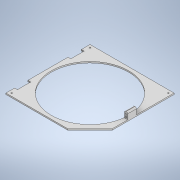
# Autodesk Inventor part: Box_Walls_2
Saved by Autodesk Inventor 2022 (Build 260153000, 153)
## iProperties
Created: 2023-02-27
Part Number: Box_Walls_2
Material: Generic
Document SubType Name: Modeling
Designer: zarek
Density: 1 g/cm^3
Appearance: Default
Author: zarek
Autodesk Inventor part; units mm, degrees
ref_plane "YZ Plane" through (0, 0, 0) normal (1, 0, 0) x (0, 1, 0)
ref_plane "XZ Plane" through (0, 0, 0) normal (0, 1, 0) x (-1, 0, 0)
ref_plane "XY Plane" through (0, 0, 0) normal (0, 0, 1) x (1, 0, 0)
sketch "Sketch1" plane through (0, 0, 0) normal (0, 1, 0) x (-1, 0, 0)
  line L0 (101.6, -101.6) -> (-101.6, -101.6)
  line L1 (-101.6, -101.6) -> (-101.6, 101.6)
  line L2 (-101.6, 101.6) -> (101.6, 101.6)
  line L3 (101.6, 101.6) -> (101.6, -101.6)
  line L4 (96.6, -96.6) -> (-96.6, -96.6)
  line L5 (-96.6, -96.6) -> (-96.6, 96.6)
  line L6 (-96.6, 96.6) -> (96.6, 96.6)
  line L7 (96.6, 96.6) -> (96.6, -96.6)
  line L8 (101.6, 101.6) -> (-40.4, 101.6)
  circle A0 centre (0, 0) radius 88.9
  circle A1 centre (0, 0) radius 109.3376
  line L9 (-40.4, 101.6) -> (-101.6, 40.4)
  line L10 (-45.4, 101.6) -> (-101.6, 45.4)
  line L11 (96.6, 96.6) -> (96.6, 101.6)
  line L12 (-45.4, 101.6) -> (-35.4, 101.6)
  line L13 (-35.4, 101.6) -> (-35.4, 96.6)
  line L14 (-35.4, 96.6) -> (-45.4, 96.6)
  line L15 (-45.4, 96.6) -> (-45.4, 101.6)
  circle A2 centre (0, 0) radius 111.3376
  point P0 (96.6, 51.2168)
  point P1 (101.6, 40.4)
  point P2 (101.6, -40.4)
  point P3 (96.6, -51.2168)
  point P4 (-96.6, 45.4)
  point P5 (-45.4, 96.6)
  dimension "d0" = 203.2
  dimension "d1" = 203.2
  dimension "d2" = 101.6
  dimension "d3" = 101.6
  dimension "d4" = 5
  dimension "d5" = 5
  dimension "d6" = 5
  dimension "d7" = 5
  dimension "d10" = 142
  dimension "d12" = 61.2
  dimension "d14" = 177.8
  dimension "d15" = 5
  dimension "d16" = 5
  dimension "d17" = 10
  dimension "d34" = 2
  constraints: 32 end point, 7 parallel, 6 point on line, 4 perpendicular, 3 centre point, 3 coincident, 3 horizontal, 2 point on circle
  measures "d0" distance between parallel lines of L2 L0
  measures "d1" distance between parallel lines of L1 L3
  measures "d2" distance from line of L0 point (0, 0)
  measures "d3" distance from line of L1 point (0, 0)
  measures "d4" distance between parallel lines of L4 L0
  measures "d5" distance between parallel lines of L1 L5
  measures "d6" distance between parallel lines of L2 L6
  measures "d7" distance between parallel lines of L3 L7
  measures "d10" distance of L2.end L8.end
  measures "d12" distance from line of L1 L8.end
  measures "d14" diameter of A0
  measures "d15" distance of L10.end L9.end
  measures "d16" distance of L10.start L8.end
  measures "d17" distance of L13.end L14.end
  measures "d34" radial gap between concentric circles of A1 A2
extrude "Extrusion1" add sketch "Sketch1" along normal blind 3 contours A2 L7 L4 | L4 A1 L7 A2 | L4 A1 L5 L9 L6 L7 | A2 L5 A1 L4 | L4 L5 A2 | A1 L6 A2 L7 | A2 L6 L7
sketch "Sketch5" plane through (0, 3, 0) normal (0, 1, 0) x (1, 0, 0)
  line L0 (-96.6, -96.6) -> (45.4, -96.6) projected
  circle A0 centre (0, 0) radius 88.9 projected
  line L1 (96.6, -45.4) -> (96.6, 96.6) projected
  line L2 (96.6, 0) -> (89.1, 0)
  line L3 (89.1, 0) -> (89.1, 10)
  line L4 (89.1, 10) -> (96.6, 10)
  line L5 (96.6, 10) -> (96.6, 0)
  line L6 (89.1, 0) -> (96.6, 0)
  line L7 (96.6, 0) -> (96.6, -10)
  line L8 (96.6, -10) -> (89.1, -10)
  line L9 (89.1, -10) -> (89.1, 0)
  line L10 (0, 0) -> (96.6, 0)
  point P0 (10, -96.6)
  dimension "d52" = 7.5
  dimension "d53" = 7.5
  dimension "d54" = 10
  dimension "d55" = 10
  constraints: 18 end point, 4 parallel, 3 horizontal, 2 perpendicular, 2 point on line
  measures "d52" distance of L3.end L4.end
  measures "d53" distance of L7.end L8.end
  measures "d54" distance between parallel lines of L6 L4
  measures "d55" distance between parallel lines of L10 L8
extrude "Extrusion4" add sketch "Sketch5" along normal blind 15 contours L3 L4 L1 L2 | L2 L1 L8 L9
sketch "Sketch7" plane through (89.1, 3, 10) normal (0, 0, 1) x (1, 0, 0)
  line L0 (2, 10) -> (5.5, 10)
  line L1 (5.5, 10) -> (5.5, 3)
  line L2 (5.5, 3) -> (2, 3)
  line L3 (2, 3) -> (2, 10)
  line L4 (7.5, 0) -> (7.5, 15)
  line L5 (0, 0) -> (0, 15)
  line L6 (0, 15) -> (7.5, 15)
  point P0 (-89.1, -3)
  dimension "d56" = 3.5
  dimension "d57" = 2
  dimension "d58" = 2
  dimension "d59" = 5
  dimension "d60" = 7
  constraints: 14 end point, 2 parallel, 1 horizontal, 1 perpendicular
  measures "d56" distance of L1.end L2.end
  measures "d57" distance between parallel lines of L4 L1
  measures "d58" distance between parallel lines of L5 L3
  measures "d59" distance between parallel lines of L0 L6
  measures "d60" distance between parallel lines of L2 L0
extrude "Extrusion6" cut sketch "Sketch7" against normal through all
fillet "Fillet7" radius 3.175 2 edges at (96.6, 18, 0) (89.1, 18, 0)
sketch "Sketch8" plane through (0, 3, 0) normal (0, 1, 0) x (1, 0, 0)
  arc A0 (-101.6, -98.425) -> (-98.425, -101.6) centre (-98.425, -98.425) ccw
  line L0 (44.0849, 101.6) -> (-98.425, 101.6)
  line L1 (-101.6, 98.425) -> (-101.6, -98.425)
  line L2 (-101.6, -46.1) -> (-101.6, -76.6)
  line L3 (-96.6, -96.6) -> (-96.6, 96.6)
  line L4 (-96.6, -46.1) -> (-96.6, -76.6)
  line L5 (-101.6, -76.6) -> (-96.6, -76.6)
  line L6 (-101.6, -46.1) -> (-96.6, -46.1)
  line L7 (-98.425, -101.6) -> (101.6, -101.6)
  line L8 (0, 0) -> (-101.6, 0)
  line L9 (-101.6, 46.1) -> (-101.6, 76.6)
  line L10 (-96.6, 46.1) -> (-96.6, 76.6)
  line L11 (-101.6, 76.6) -> (-96.6, 76.6)
  line L12 (-101.6, 46.1) -> (-96.6, 46.1)
  line L13 (-96.6, -76.6) -> (-90.1, -76.6)
  line L14 (-90.1, -76.6) -> (-90.1, -46.1)
  line L15 (-90.1, -46.1) -> (-96.6, -46.1)
  line L16 (-96.6, -46.1) -> (-96.6, -76.6)
  arc A1 (-98.425, 101.6) -> (-101.6, 98.425) centre (-98.425, 98.425) ccw
  line L17 (-101.6, 46.1) -> (-101.6, 76.6)
  line L18 (-96.6, 46.1) -> (-96.6, 76.6)
  line L19 (-101.6, 76.6) -> (-96.6, 76.6)
  line L20 (-101.6, 46.1) -> (-96.6, 46.1)
  line L21 (-96.6, 76.6) -> (-90.1, 76.6)
  line L22 (-90.1, 76.6) -> (-90.1, 46.1)
  line L23 (-90.1, 46.1) -> (-96.6, 46.1)
  line L24 (-96.6, 46.1) -> (-96.6, 76.6)
  point P0 (-98.425, 98.425)
  point P1 (46.1, 101.6)
  point P2 (46.1, 96.6)
  point P3 (76.6, 96.6)
  point P4 (76.6, 101.6)
  point P5 (-46.1, 96.6)
  dimension "d64" = 30.5
  dimension "d65" = 25
  dimension "d66" = 6.5
  constraints: 50 end point, 10 symmetric about line, 4 point on circle, 3 parallel, 3 point on line, 2 centre point, 2 perpendicular, 1 horizontal, 1 midpoint, 1 other
  measures "d64" distance between parallel lines of L5 L6
  measures "d65" distance between parallel lines of L5 L7
  measures "d66" distance between parallel lines of L14 L3
extrude "Extrusion7" cut sketch "Sketch8" against normal through all contours L21 L22 L23 L3 | L15 L14 L13 L3
sketch "Sketch10" plane through (0, 0, 0) normal (0, -1, 0) x (1, 0, 0)
  line L0 (-90, -90) -> (-90, 90)
  line L1 (-90, 90) -> (90, 90)
  line L2 (90, 90) -> (90, -90)
  line L3 (90, -90) -> (-90, -90)
  circle A0 centre (-90, -90) radius 1
  circle A1 centre (-90, 90) radius 1
  circle A2 centre (90, -90) radius 1
  point P0 (0, 0)
  point P1 (0, 0)
  dimension "d76" = 90
  dimension "d77" = 90
  dimension "d78" = 90
  dimension "d79" = 90
  dimension "d80" = 2
  dimension "d81" = 2
  dimension "d82" = 2
  constraints: 8 end point, 3 centre point, 3 coincident, 2 parallel, 1 perpendicular
  measures "d76" distance from line of point (0, 0) L0
  measures "d77" distance from line of point (0, 0) L3
  measures "d78" distance from line of point (0, 0) L1
  measures "d79" distance from line of L2 point (0, 0)
  measures "d80" diameter of A0
  measures "d81" diameter of A1
  measures "d82" diameter of A2
hole "Hole1" at (90, 0, -90) at (-90, 0, 90) at (-90, 0, -90) direction (0, 1, 0) diameter 2.85 depth 4 tip angle 118 countersink diameter 5.2 countersink angle 90 thread size "M3.5x0.6" class "6H" standard "ANSI Metric M Profile"
equation "\"d1\" = d0"
equation "\"d2\" = 0.5 * d0"
equation "\"d3\" = 0.5 * d0"
body "Solid1"
